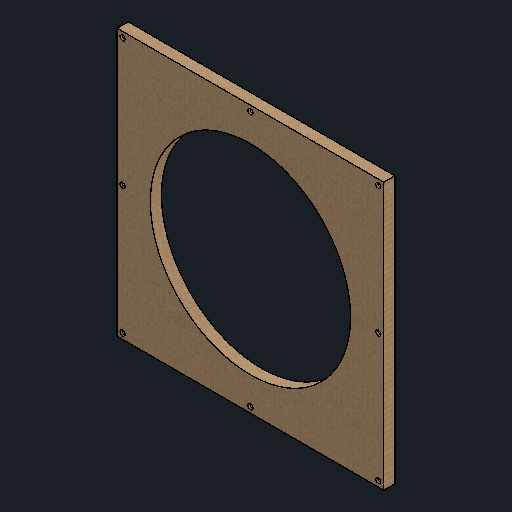
# Autodesk Inventor part: Part1
Saved by Autodesk Inventor 2026.2 (Build 302298000, 298)
## iProperties
Created: 2026-06-15
Part Number: Part1
Material: MDF Medium Density Fiberboard
Document SubType Name: Modeling
Designer: JoshuaEah
Density: 0.8 g/cm^3
Appearance: Cardboard - Corrugated
Author: JoshuaEah
Autodesk Inventor part; units mm, degrees
ref_plane "YZ Plane" through (0, 0, 0) normal (1, 0, 0) x (0, 1, 0)
ref_plane "XZ Plane" through (0, 0, 0) normal (0, 1, 0) x (-1, 0, 0)
ref_plane "XY Plane" through (0, 0, 0) normal (0, 0, 1) x (1, 0, 0)
sketch "Sketch1" plane through (0, 0, 0) normal (0, 0, 1) x (1, 0, 0)
  line L0 (0, 0) -> (304.8, 0)
  line L1 (304.8, 0) -> (304.8, 304.8)
  line L2 (304.8, 304.8) -> (0, 304.8)
  line L3 (0, 304.8) -> (0, 0)
  circle A0 centre (152.4, 152.4) radius 114.3
  circle A1 centre (6.35, 298.45) radius 0.9922
  circle A2 centre (298.45, 298.45) radius 0.9922
  circle A3 centre (298.45, 6.35) radius 0.9922
  circle A4 centre (6.35, 6.35) radius 0.9922
  circle A5 centre (6.35, 152.4) radius 0.9922
  circle A6 centre (298.45, 152.4) radius 0.9922
  circle A7 centre (152.4, 298.45) radius 0.9922
  circle A8 centre (152.4, 6.35) radius 0.9922
  point P0 (304.8, 152.4)
  point P1 (152.4, 304.8)
  dimension "d0" = 304.8
  dimension "d1" = 228.6
  dimension "d6" = 1.9844
  dimension "d7" = 6.35
  dimension "d8" = 6.35
  dimension "d10" = 6.35
  dimension "d11" = 6.35
  constraints: 9 centre point, 8 end point, 7 equal radius, 7 horizontal alignment, 7 vertical alignment, 2 midpoint, 2 parallel, 2 perpendicular, 1 coincident, 1 horizontal
  measures "d0" distance of L1.end L2.end
  measures "d1" diameter of A0
  measures "d6" diameter of A1
  measures "d7" distance from line of L3 A1.centre
  measures "d8" distance from line of L2 A1.centre
  measures "d10" distance from line of L1 A2.centre
  measures "d11" distance from line of L0 A3.centre
extrude "Extrusion1" add sketch "Sketch1" against normal blind 12.7 contours L3 L2 L1 L0 | A1 | A2 | A3 | A4 | A5 | A6 | A7 | A8
hole "Hole1" at (6.35, 298.45, 0) at (298.45, 298.45, 0) at (298.45, 6.35, 0) at (6.35, 6.35, 0) at (152.4, 298.45, 0) at (152.4, 6.35, 0) at (298.45, 152.4, 0) at (6.35, 152.4, 0) direction (0, 0, -1) diameter 3.2766 end through all countersink diameter 5.715 countersink angle 82 clearance for "Flat Head Machine Screw (82)" size "#4" standard "Ansi Unified Screw Threads"
equation "\"d10\" = d7"
equation "\"d11\" = d8"
body "Solid1"
